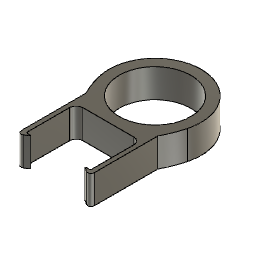
keycap-puller-v3 (Autodesk Fusion 360 design; units mm, degrees)
Autodesk Fusion 360 part; units mm, degrees
sketch "Sketch1" plane through (0, 0, 0) normal (0, 0, 1) x (1, 0, 0)
  line L0 (0, 0) -> (18, 0)
  line L1 (0, 0) -> (0, -15)
  line L2 (18, 0) -> (18, -15)
  line L3 (0, -15) -> (1.7321, -14)
  line L4 (0, -15) -> (2, -15) construction
  line L5 (1.7321, -14) -> (0, -14)
  line L6 (18, -15) -> (16.2679, -14)
  line L7 (18, -15) -> (20, -15) construction
  line L8 (16.2679, -14) -> (18, -14)
  line L9 (0, -15) -> (-1.9645, -14.6248)
  line L10 (-1.9645, -14.6248) -> (-1.9645, 3.9225)
  line L11 (18, -15) -> (19.9559, -14.5824)
  line L12 (19.9559, -14.5824) -> (19.9559, 3.6155)
  circle A0 centre (9.0998, 12.9334) radius 10
  circle A1 centre (9.0998, 12.9334) radius 12.8772
  line L13 (-1.9645, 3.9225) -> (-3.4142, 9.8967)
  line L14 (19.9559, 3.6155) -> (21.5492, 9.6419)
  dimension "d1" = 18
  dimension "d2" = 15
  dimension "d3" = 15
  dimension "d4" = 2
  dimension "d5" = 30
  dimension "d6" = 150
  dimension "d7" = 2
  dimension "d8" = 2
  dimension "d9" = 20
  dimension "d10" = 2
  constraint coincident L0.start L1.start
  constraint horizontal L0
  constraint perpendicular L0 L1
  constraint perpendicular L0 L2
  constraint horizontal L4
  constraint coincident L1 L5.end
  constraint perpendicular L1 L5
  constraint horizontal L7
  constraint coincident L2 L8.end
  constraint perpendicular L2 L8
  constraint perpendicular L5 L10
  constraint perpendicular L7 L12
  constraint concentric A0 A1
  constraint coincident A1 L13.end
  constraint tangent A1 L13
  constraint coincident A1 L14.end
  constraint tangent A1 L14
  measures "d1" distance of L0.start L0.end
  measures "d2" distance of L0.start L1.end
  measures "d3" distance of L0.end L2.end
  measures "d4" distance of L1.end L3.end
  measures "d5" angle of L3 L4
  measures "d6" angle of L6 L7
  measures "d7" distance of L2.end L6.end
  measures "d8" distance of L1.end L9.end
  measures "d9" diameter of A0
  measures "d10" distance of L2.end L11.end
extrude "Extrude1" add sketch "Sketch1" along normal blind 8
fillet "Fillet1" radius 2.5 1 edges at (19.9559, -14.5824, 4)
fillet "Fillet2" radius 2.5 1 edges at (-1.9645, -14.6248, 4)
fillet "Fillet3" radius 1 1 edges at (-0.2235, 16.5496, 8)
fillet "Fillet4" radius 1 1 edges at (-0.2235, 16.5496, 0)
fillet "Fillet5" radius 2 1 edges at (18, 0, 4)
fillet "Fillet6" radius 2 1 edges at (0, 0, 4)
fillet "Fillet7" radius 1 1 edges at (0, -15, 4)
fillet "Fillet8" radius 1 1 edges at (18, -15, 4)
extrude "Extrude2" cut 1 faces at (19.9559, -7.168, 2.6667) along direction (-1, 0, 0) blind 0.75
extrude "Extrude3" cut 1 faces at (-1.9645, -7.0639, 2.6667) along direction (1, 0, 0) blind 0.75
fillet "Fillet9" radius 20.25 1 edges at (-1.9645, 3.9225, 4)
fillet "Fillet10" radius 23 1 edges at (19.9559, 3.6155, 4)
delete_face "DeleteFace1" 1 faces at (19.7059, -12.5598, 2.6667)
delete_face "DeleteFace2" 1 faces at (19.0612, -14.4763, 5.3333)
delete_face "DeleteFace3" [no effect]
delete_face "DeleteFace4" [no effect]
delete_face "DeleteFace5" 1 faces at (17.1632, -14.5169, 2.6667)
extrude "Extrude4" cut 1 faces at (18.5735, -13.5009, 8) along direction (0, 0, -1) blind 19
extrude "Extrude5" add sketch "Sketch1" against normal blind 8
extrude "Extrude6" cut 1 faces at (19.9559, -8.5164, -2.6667) along direction (-1, 0, 0) blind 0.75
extrude "Extrude7" cut 1 faces at (-1.9645, -8.4424, -2.6667) along direction (1, 0, 0) blind 0.75
delete_face "DeleteFace6" 1 faces at (-1.7145, -14.6248, -2.6667)
delete_face "DeleteFace7" 1 faces at (19.7059, -14.5824, -2.6667)
fillet "Fillet11" radius 27.375 2 edges at (19.9559, 3.6155, -4) (-1.9645, 3.9225, -4)
fillet "Fillet12" radius 3.125 1 edges at (18, -15, -4)
fillet "Fillet13" radius 3.625 1 edges at (0, -15, -4)
fillet "Fillet14" radius 0.625 1 edges at (-1.2145, -14.7681, -4)
fillet "Fillet15" radius 1.875 2 edges at (18, 0, -4) (0, 0, -4)
fillet "Fillet16" radius 0.125 1 edges at (16.2679, -14, -4)
fillet "Fillet17" radius 0.125 1 edges at (1.7321, -14, -4)
fillet "Fillet18" radius 0.375 2 edges at (0, -14, -4) (18, -14, -4)
fillet "Fillet19" radius 2.5 1 edges at (19.2059, -14.7425, -4)
delete_face "DeleteFace8" 1 faces at (-1.2116, -14.246, -5.3333)
delete_face "DeleteFace9" 1 faces at (18.5679, -14.8177, -2.6667)
delete_face "DeleteFace10" 1 faces at (-1.0513, -14.7885, -5.3333)
delete_face "DeleteFace11" 1 faces at (19.2039, -14.4571, -2.6667)
fillet "Fillet20" radius 0.875 2 edges at (-1.2145, -15.7012, -4) (19.2059, -15.6962, -4)
